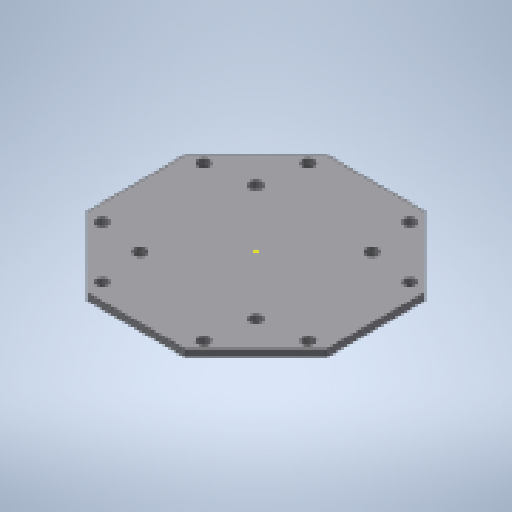
# Autodesk Inventor part: 上板
Saved by Autodesk Inventor 2025.2 (Build 292293000, 293)
## iProperties
Created: 2026-03-19
Part Number: 上板
Material: 常规
Document SubType Name: Modeling
Designer: BO‘S_SLAVE
Density: 1 g/cm^3
Appearance: 默认
Author: BO‘S_SLAVE
Autodesk Inventor part; units mm, degrees
ref_plane "YZ Plane" through (0, 0, 0) normal (1, 0, 0) x (0, 1, 0)
ref_plane "XZ Plane" through (0, 0, 0) normal (0, 1, 0) x (-1, 0, 0)
ref_plane "XY Plane" through (0, 0, 0) normal (0, 0, 1) x (1, 0, 0)
sketch "草图1" plane through (0, 0, 0) normal (0, 1, 0) x (-1, 0, 0)
  line L0 (25.1023, 25.1023) -> (-25.1023, 25.1023)
  line L1 (-25.1023, 25.1023) -> (-25.1023, -25.1023)
  line L2 (-25.1023, -25.1023) -> (25.1023, -25.1023)
  line L3 (25.1023, -25.1023) -> (25.1023, 25.1023)
  line L4 (25.1023, 25.1023) -> (-25.1023, -25.1023)
  line L5 (25.1023, -25.1023) -> (-25.1023, 25.1023)
  line L6 (-14.4957, 35.7089) -> (-35.7089, 14.4957)
  line L7 (-35.7089, -14.4957) -> (-14.4957, -35.7089)
  line L8 (14.4957, -35.7089) -> (35.7089, -14.4957)
  line L9 (35.7089, 14.4957) -> (14.4957, 35.7089)
  line L10 (14.4957, 35.7089) -> (-14.4957, 35.7089)
  line L11 (35.7089, 14.4957) -> (35.7089, -14.4957)
  line L12 (14.4957, -35.7089) -> (-14.4957, -35.7089)
  line L13 (-35.7089, -14.4957) -> (-35.7089, 14.4957)
  circle A0 centre (30.7591, 15.2028) radius 1.65
  circle A1 centre (17.3241, 17.3241) radius 1.65
  circle A2 centre (15.2028, 30.7591) radius 1.65
  circle A3 centre (-15.2028, 30.7591) radius 1.65
  circle A4 centre (-17.3241, 17.3241) radius 1.65
  circle A5 centre (-30.7591, 15.2028) radius 1.65
  circle A6 centre (-30.7591, -15.2028) radius 1.65
  circle A7 centre (-17.3241, -17.3241) radius 1.65
  circle A8 centre (-15.2028, -30.7591) radius 1.65
  circle A9 centre (15.2028, -30.7591) radius 1.65
  circle A10 centre (17.3241, -17.3241) radius 1.65
  circle A11 centre (30.7591, -15.2028) radius 1.65
  point P0 (0, 0)
  point P1 (0, 0)
  point P2 (-25.1023, -25.1023)
  point P3 (25.1023, 25.1023)
  dimension "d0" = 71
  dimension "d1" = 30
  dimension "d2" = 45
  dimension "d5" = 360
  dimension "d12" = 3.3
  dimension "d13" = 3
  dimension "d14" = 11
  dimension "d15" = 3.3
  dimension "d16" = 11
  dimension "d19" = 360
  constraints: 28 end point, 12 centre point, 6 perpendicular, 2 midpoint, 2 parallel, 1 coincident, 1 horizontal, 1 point on line, 1 symmetric about line, 43 other
  measures "d0" distance of L2.end L0.end
  measures "d1" distance of L6.start L6.end
  measures "d2" angle of L6 L1
  measures "d12" diameter of A0
  measures "d13" distance from line of L9 A0.centre
  measures "d14" distance from line of L4 A0.centre
  measures "d15" diameter of A1
  measures "d16" distance from line of L9 A1.centre
extrude "拉伸1" add sketch "草图1" along normal blind 2 contours L4 A1 L5 A4 L0 | L9 L11 L8 L3 | L3 L5 A10 L4 A1 | L0 L6 L10 L9 | L5 A4 L4 A7 L1 | L1 L7 L13 L6 | L8 L12 L7 L2 | L2 L4 A7 L5 A10
sketch "草图2" plane through (0, 2, 0) normal (0, 1, 0) x (1, 0, 0)
  point P0 (0, 0)
